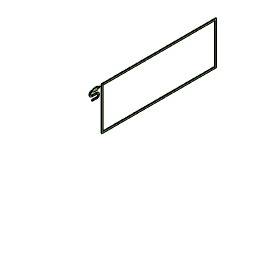
Schrift_Seitenteil_links (Autodesk Fusion 360 design; units mm, degrees)
Autodesk Fusion 360 part; units mm, degrees
note: some values were not read from the file. Set by a fixed rule: which sketch regions a step uses.
sketch "Skizze1" plane through (70, 0, 0) normal (1, 0, 0) x (0, 1, 0)
  line L0 (60.6546, 145.6) -> (60.6546, 100.6)
  line L1 (60.6546, 100.6) -> (-59.6, 100.6)
  line L2 (-59.6, 100.6) -> (-59.6, 145.6)
  line L3 (-59.6, 145.6) -> (60.6546, 145.6)
  line L4 (-74.1, 83.1) -> (74.1, 83.1)
  line L5 (74.1, 83.1) -> (74.1, 152.2)
  arc A0 (74.1, 152.2) -> (73.2, 153.1) centre (73.2, 152.2) ccw
  line L6 (73.2, 153.1) -> (-73.2, 153.1)
  arc A1 (-73.2, 153.1) -> (-74.1, 152.2) centre (-73.2, 152.2) ccw
  line L7 (-74.1, 152.2) -> (-74.1, 83.1)
  line L8 (-58.1, 102.1) -> (-58.1, 144.1)
  line L9 (-58.1, 144.1) -> (59.1546, 144.1)
  line L10 (59.1546, 144.1) -> (59.1546, 102.1)
  line L11 (59.1546, 102.1) -> (-58.1, 102.1)
  line L12 (-59.6, 100.6) -> (60.6546, 100.6)
  line L13 (60.6546, 100.6) -> (60.6546, 145.6)
  line L14 (60.6546, 145.6) -> (-59.6, 145.6)
  line L15 (-59.6, 145.6) -> (-59.6, 100.6)
  arc A2 (-69.6, 144.7) -> (-69.6, 139.3) centre (-69.6, 142) ccw
  line L16 (-69.6, 144.7) -> (-68.6, 144.7)
  line L17 (-68.6, 144.7) -> (-68.6, 144.85)
  line L18 (-68.6, 144.85) -> (-67.85, 145.6)
  line L19 (-67.85, 145.6) -> (-63.6, 145.6)
  line L20 (-63.6, 145.6) -> (-63.6, 144.6)
  line L21 (-63.6, 144.6) -> (-61.6, 144.6)
  line L22 (-61.6, 143.6) -> (-63.6, 143.6)
  line L23 (-63.6, 143.6) -> (-63.6, 142.6)
  line L24 (-63.6, 142.6) -> (-67.85, 142.6)
  line L25 (-67.85, 142.6) -> (-68.6, 143.35)
  line L26 (-68.6, 143.35) -> (-68.6, 143.5)
  line L27 (-68.6, 143.5) -> (-69.6, 143.5)
  arc A3 (-69.6, 143.5) -> (-69.6, 140.5) centre (-69.6, 142) ccw
  line L28 (-69.6, 140.5) -> (-64.6, 140.5)
  arc A4 (-64.6, 135.1) -> (-64.6, 140.5) centre (-64.6, 137.8) ccw
  line L29 (-64.6, 135.1) -> (-69.6, 135.1)
  line L30 (-69.6, 135.1) -> (-69.6, 136.3)
  line L31 (-69.6, 136.3) -> (-64.6, 136.3)
  arc A5 (-64.6, 136.3) -> (-64.6, 139.3) centre (-64.6, 137.8) ccw
  line L32 (-64.6, 139.3) -> (-69.6, 139.3)
  arc A6 (-61.6, 143.6) -> (-61.6, 144.6) centre (-61.6, 144.1) ccw
  arc A7 (-61.6, 143.6) -> (-61.6, 144.6) centre (-61.6, 144.1) ccw
  line L33 (-61.6, 143.6) -> (-63.6, 143.6)
  line L34 (-63.6, 143.6) -> (-63.6, 142.6)
  line L35 (-63.6, 142.6) -> (-67.85, 142.6)
  line L36 (-67.85, 142.6) -> (-68.6, 143.35)
  line L37 (-68.6, 143.35) -> (-68.6, 143.5)
  line L38 (-68.6, 143.5) -> (-69.6, 143.5)
  arc A8 (-69.6, 143.5) -> (-69.6, 140.5) centre (-69.6, 142) ccw
  line L39 (-69.6, 140.5) -> (-64.6, 140.5)
  arc A9 (-64.6, 135.1) -> (-64.6, 140.5) centre (-64.6, 137.8) ccw
  line L40 (-64.6, 135.1) -> (-69.6, 135.1)
  line L41 (-69.6, 135.1) -> (-69.6, 136.3)
  line L42 (-69.6, 136.3) -> (-64.6, 136.3)
  arc A10 (-64.6, 136.3) -> (-64.6, 139.3) centre (-64.6, 137.8) ccw
  line L43 (-64.6, 139.3) -> (-69.6, 139.3)
  arc A11 (-69.6, 144.7) -> (-69.6, 139.3) centre (-69.6, 142) ccw
  line L44 (-69.6, 144.7) -> (-68.6, 144.7)
  line L45 (-68.6, 144.7) -> (-68.6, 144.85)
  line L46 (-68.6, 144.85) -> (-67.85, 145.6)
  line L47 (-67.85, 145.6) -> (-63.6, 145.6)
  line L48 (-63.6, 145.6) -> (-63.6, 144.6)
  line L49 (-63.6, 144.6) -> (-61.6, 144.6)
  line L50 (60.6546, 145.6) -> (60.6546, 100.6)
  line L51 (60.6546, 100.6) -> (-59.6, 100.6)
  line L52 (-59.6, 100.6) -> (-59.6, 145.6)
  line L53 (-59.6, 145.6) -> (60.6546, 145.6)
  line L54 (-74.1, 83.1) -> (74.1, 83.1)
  line L55 (74.1, 83.1) -> (74.1, 152.2)
  arc A12 (74.1, 152.2) -> (73.2, 153.1) centre (73.2, 152.2) ccw
  line L56 (73.2, 153.1) -> (-73.2, 153.1)
  arc A13 (-73.2, 153.1) -> (-74.1, 152.2) centre (-73.2, 152.2) ccw
  line L57 (-74.1, 152.2) -> (-74.1, 83.1)
extrude "Extrusion1" add sketch "Skizze1" against normal up to surface (0.6 mm away) contours L0 L1 L2 L3 L12 L13 L14 L15 L50 L51 L52 L53 | A2 L16 L17 L18 L19 L20 L21 L22 L23 L24 L25 L26 L27 A3 L28 A4 L29 L30 L31 A5 L32 A6 A7 L33 L34 L35 L36 L37 L38 A8 L39 A9 L40 L41 L42 A10 L43 A11 L44 L45 L46 L47 L48 L49 makes body 1 at (70, -19.0151, 145.1) makes body 2 at (70, -66.4333, 144.2667)
